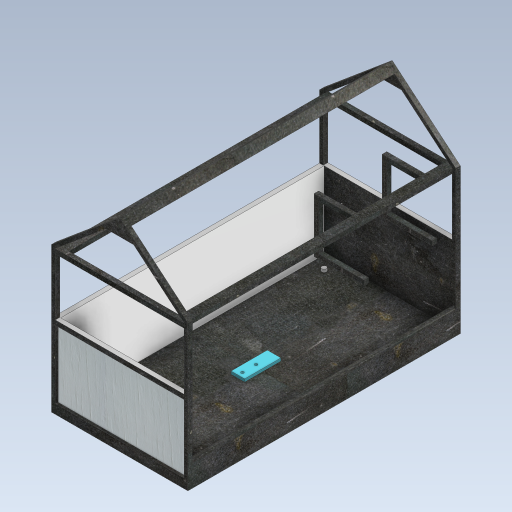
# Autodesk Inventor part: estructuragen
Saved by Autodesk Inventor 2023 (Build 270158000, 158)
## iProperties
Created: 2023-03-08
Part Number: estructuragen
Material: Steel
Document SubType Name: Modeling
Designer: santi
Density: 7.85 g/cm^3
Appearance: Plate
Author: santi
Autodesk Inventor part; units mm, degrees
ref_plane "YZ Plane" through (0, 0, 0) normal (1, 0, 0) x (0, 1, 0)
ref_plane "XZ Plane" through (0, 0, 0) normal (0, 1, 0) x (-1, 0, 0)
ref_plane "XY Plane" through (0, 0, 0) normal (0, 0, 1) x (1, 0, 0)
sketch "Sketch1" plane through (0, 0, 0) normal (0, 1, 0) x (-1, 0, 0)
  line L0 (0, 0) -> (150, 0)
  line L1 (150, 0) -> (150, -300)
  line L2 (150, -300) -> (0, -300)
  line L3 (0, -300) -> (0, 0)
  dimension "d0" = 150
  dimension "d1" = 300
  constraints: 8 end point, 2 parallel, 1 horizontal, 1 perpendicular
  measures "d0" distance of L1.end L2.end
  measures "d1" distance of L0.end L1.end
extrude "Extrusion1" add sketch "Sketch1" along normal blind 5
sketch "Sketch2" plane through (0, 5, 0) normal (0, 1, 0) x (1, 0, 0)
  line L0 (-150, 0) -> (0, 0) projected
  line L1 (0, 300) -> (-150, 300) projected
  line L2 (0, 0) -> (-150, 0)
  line L3 (-150, 0) -> (-150, 300)
  line L4 (-150, 300) -> (0, 300)
  line L5 (0, 300) -> (0, 0)
  line L6 (-145, 295) -> (-145, 5)
  line L7 (-145, 5) -> (-5, 5)
  line L8 (-5, 5) -> (-5, 295)
  line L9 (-5, 295) -> (-145, 295)
  line L10 (-5, 5) -> (-145, 5)
  line L11 (-145, 5) -> (-145, 295)
  line L12 (-145, 295) -> (-5, 295)
  line L13 (-5, 295) -> (-5, 5)
  line L14 (0, 0) -> (-150, 0)
  line L15 (-150, 0) -> (-150, 300)
  line L16 (-150, 300) -> (0, 300)
  line L17 (0, 300) -> (0, 0)
  point P0 (0, 300)
  point P1 (-150, 0)
  dimension "d4" = 5
  constraints: 32 end point, 8 parallel, 4 perpendicular, 3 horizontal, 3 other
  measures "d4" distance between parallel lines of L3 L6
extrude "Extrusion2" add sketch "Sketch2" along normal blind 5
sketch "Sketch3" plane through (-150, 0, 0) normal (0, 0, 1) x (1, 0, 0)
  line L0 (150, 10) -> (0, 10) projected
  line L1 (0, 10) -> (150, 10)
  line L2 (0, 10) -> (150, 10)
  line L3 (150, 10) -> (150, 160)
  line L4 (0, 10) -> (0, 160)
  line L5 (0, 160) -> (75, 222.9325)
  line L6 (75, 222.9325) -> (150, 160)
  line L7 (146, 10) -> (146, 158.1348)
  line L8 (146, 158.1348) -> (75, 217.7108)
  line L9 (75, 217.7108) -> (4, 158.1348)
  line L10 (4, 158.1348) -> (4, 10)
  line L11 (5, 10) -> (145, 10) projected
  line L12 (5, 10) -> (0, 10)
  line L13 (145, 10) -> (150, 10)
  point P0 (150, 0)
  dimension "d7" = 150
  dimension "d8" = 150
  dimension "d9" = 130
  dimension "d10" = 130
  dimension "d11" = 4
  constraints: 24 end point, 1 horizontal, 1 perpendicular, 1 vertical, 3 other
  measures "d7" distance of L0.start L3.end
  measures "d8" distance of L0.end L4.end
  measures "d9" angle of L4 L5
  measures "d10" angle of L6 L3
  measures "d11" distance between parallel lines of L6 L8
extrude "Extrusion3" add sketch "Sketch3" against normal blind 5 contours L0 L7 L8 L9 L10 L4 L5 L6 L3
ref_plane "Work Plane1" through (-150, 0, -150) normal (0, 0, 1) x (1, 0, 0)
mirror "Mirror1" about plane through (-150, 0, -150) normal (0, 0, 1) of "Extrusion3"
sketch "Sketch4" plane through (-150, 0, -5) normal (0, 0, -1) x (-1, 0, 0)
  line L0 (-145, 10) -> (-5, 10) projected
  line L1 (-5, 10) -> (-3, 10)
  line L2 (-3, 10) -> (-3, 90)
  line L3 (-3, 90) -> (-5, 90)
  line L4 (-5, 90) -> (-5, 10)
  point P0 (-150, 0)
  dimension "d14" = 2
  dimension "d15" = 80
  constraints: 8 end point, 2 parallel, 1 horizontal, 1 perpendicular
  measures "d14" distance of L3.end L2.end
  measures "d15" distance of L2.end L1.end
extrude "Extrusion4" add sketch "Sketch4" along normal up to surface (290 mm away)
sketch "Sketch5" plane through (-4, 10, -300) normal (-1, 0, 0) x (0, 0, 1)
  line L0 (5, 0) -> (5, 80) projected
  line L1 (5, 0) -> (3, 0)
  line L2 (3, 0) -> (3, 80)
  line L3 (3, 80) -> (5, 80)
  line L4 (5, 80) -> (5, 0)
  point P0 (300, -10)
  point P1 (5, 80)
  dimension "d18" = 2
  dimension "d40" = 80
  constraints: 8 end point, 2 parallel, 1 horizontal, 1 perpendicular
  measures "d18" distance of L2.end L3.end
  measures "d40" distance of L1.end L2.end
extrude "Extrusion5" add sketch "Sketch5" along normal up to surface (142 mm away)
mirror "Mirror2" about plane through (-150, 0, -150) normal (0, 0, 1) of "Extrusion5"
sketch "Sketch12" plane through (-146, 10, 0) normal (1, 0, 0) x (0, 0, -1)
  line L0 (3, 0) -> (3, 80) construction
  line L1 (3, 80) -> (3, 75)
  line L2 (3, 75) -> (0, 75)
  line L3 (0, 0) -> (0, 148.1348) construction
  line L4 (0, 75) -> (0, 80)
  line L5 (0, 80) -> (3, 80)
  point P0 (0, -10)
  dimension "d43" = 5
  constraints: 8 end point, 2 perpendicular, 2 point on line, 1 vertical
  measures "d43" distance of L0.end L1.end
extrude "Extrusion10" add sketch "Sketch12" along normal up to surface (142 mm away)
mirror "Mirror4" about plane through (-150, 0, -150) normal (0, 0, 1) of "Extrusion10"
sketch "Sketch13" plane through (-5, 5, -5) normal (0, 0, -1) x (-1, 0, 0)
  line L0 (141, 85) -> (-1, 85) construction
  line L1 (145, -5) -> (145, 155) construction
  line L2 (141, 85) -> (145, 85)
  line L3 (145, 85) -> (145, 80)
  line L4 (145, 80) -> (141, 80)
  line L5 (141, 80) -> (141, 85)
  point P0 (-5, -5)
  dimension "d46" = 5
  constraints: 8 end point, 2 parallel, 1 horizontal, 1 perpendicular, 1 point on line
  measures "d46" distance of L2.end L3.end
extrude "Extrusion11" add sketch "Sketch13" along normal up to surface (290 mm away)
chamfer "Chamfer1" distance 20 angle 45 1 edges at (-75, 217.7108, -297.5)
chamfer "Chamfer2" distance 20 angle 45 1 edges at (-75, 217.7108, -2.5)
sketch "Sketch16" plane through (-150, 0, 0) normal (0, 0, 1) x (1, 0, 0)
  circle A0 centre (75, 214.8551) radius 1.5
  line L0 (90.3209, 204.8551) -> (59.6791, 204.8551) projected
  point P0 (150, 0)
  point P1 (75, 204.8551)
  point P2 (75, 222.9325)
  dimension "d62" = 3
  dimension "d63" = 10
  constraints: 1 centre point, 1 midpoint, 1 vertical alignment
  measures "d62" diameter of A0
  measures "d63" distance of point (75, 204.855) A0.centre
extrude "Extrusion14" cut sketch "Sketch16" against normal blind 310.0375
sketch "Sketch17" plane through (-145, 5, -295) normal (0, 0, 1) x (1, 0, 0)
  line L0 (145, 155) -> (70, 217.9325) construction
  line L1 (70, 217.9325) -> (62.3396, 211.5046)
  line L2 (70, 217.9325) -> (-5, 155) construction
  line L3 (62.3396, 211.5046) -> (77.6604, 211.5046)
  line L4 (77.6604, 211.5046) -> (70, 217.9325)
  point P0 (145, -5)
  dimension "d70" = 10
  constraints: 6 end point, 2 point on line, 1 horizontal
  measures "d70" distance of L0.end L1.end
extrude "Extrusion15" add sketch "Sketch17" along normal up to surface (290 mm away)
sketch "Sketch19" plane through (-146, 158.1348, -295) normal (1, 0, 0) x (0, 0, -1)
  line L0 (5, 1.8652) -> (0, 1.8652) construction
  line L1 (0, 1.8652) -> (0, 58.3698) construction
  line L2 (0, 1.8652) -> (5, 1.8652) construction
  line L3 (0, 1.8652) -> (0, -0.1348) construction
  line L4 (0, -68.1348) -> (0, 1.8652) construction
  line L5 (0, -0.1348) -> (5, -0.1348) construction
  line L6 (5, -158.1348) -> (5, 1.8652) construction
  line L7 (5, 64.7977) -> (5, 1.8652) construction
  line L8 (5, -0.1348) -> (5, 1.8652) construction
  line L9 (0, -0.1348) -> (5, -0.1348)
  line L10 (5, -0.1348) -> (5, -5.1348)
  line L11 (5, -5.1348) -> (0, -5.1348)
  line L12 (0, -5.1348) -> (0, -0.1348)
  point P0 (-295, -158.1348)
  dimension "d77" = 2
  dimension "d78" = 5
  constraints: 16 end point, 3 point on line, 2 horizontal, 2 parallel, 2 perpendicular, 1 vertical
  measures "d77" distance of L0.end L3.end
  measures "d78" distance of L9.end L10.end
extrude "Extrusion17" add sketch "Sketch19" along normal up to surface (142 mm away)
mirror "Mirror5" about plane through (-150, 0, -150) normal (0, 0, 1) of "Extrusion17"
sketch "Sketch20" plane through (-5, 5, -5) normal (0, 0, -1) x (-1, 0, 0)
  line L0 (141, 153) -> (-1, 153) construction
  line L1 (141, 148) -> (-1, 148) construction
  line L2 (-1, 153) -> (9, 153)
  line L3 (9, 153) -> (9, 148)
  line L4 (9, 148) -> (-1, 148)
  line L5 (-1, 148) -> (-1, 153)
  line L6 (131, 148) -> (141, 148)
  line L7 (141, 148) -> (141, 153)
  line L8 (141, 153) -> (131, 153)
  line L9 (131, 153) -> (131, 148)
  point P0 (-5, -5)
  dimension "d81" = 10
  dimension "d84" = 10
  dimension "d85" = 142
  constraints: 16 end point, 4 parallel, 3 point on line, 2 horizontal, 2 perpendicular
  measures "d81" distance of L3.end L4.end
  measures "d84" distance of L8.end L7.end
  measures "d85" distance of L6.end L1.end
extrude "Extrusion18" add sketch "Sketch20" along normal up to surface (290 mm away)
sketch "Sketch21" plane through (-14, 153, -295) normal (-1, 0, 0) x (0, 0, 1)
  line L0 (290, 5) -> (0, 5) construction
  line L1 (290, 0) -> (0, 0) construction
  line L2 (20, 5) -> (25, 5)
  line L3 (25, 5) -> (25, 0)
  line L4 (25, 0) -> (20, 0)
  line L5 (20, 0) -> (20, 5)
  line L6 (95, 5) -> (100, 5)
  line L7 (100, 5) -> (100, 0)
  line L8 (100, 0) -> (95, 0)
  line L9 (95, 0) -> (95, 5)
  line L10 (0, 0) -> (290, 0) construction
  point P0 (295, -153)
  point P1 (145, 0)
  dimension "d86" = 5
  dimension "d87" = 5
  dimension "d88" = 80
  dimension "d96" = 20
  constraints: 18 end point, 5 parallel, 4 point on line, 2 horizontal, 2 perpendicular, 1 midpoint
  measures "d86" distance of L3.end L4.end
  measures "d87" distance of L7.end L8.end
  measures "d88" distance of L7.end L4.end
  measures "d96" distance of L4.end L1.end
extrude "Extrusion19" add sketch "Sketch21" along normal blind 42
sketch "Sketch22" plane through (-146, 153, 0) normal (0, -1, 0) x (1, 0, 0)
  line L0 (90, -195) -> (90, -200) projected
  line L1 (132, -200) -> (90, -200) construction
  line L2 (90, -195) -> (95, -195)
  line L3 (95, -195) -> (95, -200)
  line L4 (95, -200) -> (90, -200)
  line L5 (90, -200) -> (90, -195)
  line L6 (90, -270) -> (90, -275) projected
  line L7 (132, -275) -> (90, -275) construction
  line L8 (90, -270) -> (95, -270)
  line L9 (95, -270) -> (95, -275)
  line L10 (95, -275) -> (90, -275)
  line L11 (90, -275) -> (90, -270)
  point P0 (146, 0)
  dimension "d92" = 5
  dimension "d93" = 5
  constraints: 16 end point, 4 parallel, 2 horizontal, 2 perpendicular, 2 point on line
  measures "d92" distance of L3.end L4.end
  measures "d93" distance of L9.end L10.end
extrude "Extrusion20" add sketch "Sketch22" along normal blind 55
sketch "Sketch23" plane through (-51, 153, -195) normal (1, 0, 0) x (0, 0, -1)
  line L0 (0, 0) -> (0, -55) construction
  line L1 (5, 5) -> (5, -55) construction
  line L2 (0, -55) -> (5, -55)
  line L3 (5, -55) -> (5, -50)
  line L4 (5, -50) -> (0, -50)
  line L5 (0, -50) -> (0, -55)
  line L6 (75, 5) -> (75, -55) construction
  line L7 (80, 0) -> (80, -55) construction
  line L8 (75, -55) -> (80, -55)
  line L9 (80, -55) -> (80, -50)
  line L10 (80, -50) -> (75, -50)
  line L11 (75, -50) -> (75, -55)
  point P0 (-195, -153)
  dimension "d97" = 5
  constraints: 16 end point, 4 parallel, 3 point on line, 2 horizontal, 2 perpendicular
  measures "d97" distance of L3.end L2.end
extrude "Extrusion21" add sketch "Sketch23" along normal blind 50
sketch "Sketch24" plane through (0, 10, 0) normal (0, 1, 0) x (1, 0, 0)
  line L0 (-5, 5) -> (-5, 295) projected
  line L1 (0, 0) -> (0, 300) construction
  line L2 (-5, 5) -> (0, 5)
  line L3 (0, 5) -> (0, 295)
  line L4 (0, 295) -> (-5, 295)
  line L5 (-5, 295) -> (-5, 5)
  constraints: 8 end point, 2 parallel, 1 horizontal, 1 perpendicular, 1 point on line
extrude "Extrusion22" add sketch "Sketch24" along normal blind 16
sketch "Sketch26" plane through (-5, 5, -5) normal (0, 0, -1) x (-1, 0, 0)
  circle A0 centre (-2.5, 22) radius 1
  line L0 (-5, 21) -> (0, 21) construction
  point P0 (-5, -5)
  point P1 (-2.5, 21)
  dimension "d103" = 2
  constraints: 1 centre point, 1 midpoint, 1 tangent, 1 vertical alignment
  measures "d103" diameter of A0
extrude "Extrusion23" cut sketch "Sketch26" against normal blind 3
mirror "Mirror6" about plane through (-150, 0, -150) normal (0, 0, 1) of "Extrusion23"
fillet "Fillet1" radius 2 1 edges at (0, 26, -150)
sketch "Sketch27" plane through (0, 5, 0) normal (0, 1, 0) x (1, 0, 0)
  line L0 (-67.5, 130) -> (-82.5, 130)
  line L1 (-82.5, 130) -> (-82.5, 170)
  line L2 (-82.5, 170) -> (-67.5, 170)
  line L3 (-67.5, 170) -> (-67.5, 130)
  line L4 (-75, 300) -> (-75, 0) construction
  line L5 (-67.5, 130) -> (-82.5, 170) construction
  line L6 (-82.5, 130) -> (-67.5, 170) construction
  circle A0 centre (-75, 135) radius 1.5
  circle A1 centre (-75, 150) radius 1.5
  point P0 (0, 0)
  dimension "d107" = 15
  dimension "d108" = 40
  dimension "d111" = 3
  dimension "d112" = 3
  dimension "d113" = 15
  dimension "d114" = 5
  constraints: 12 end point, 4 midpoint, 2 centre point, 2 parallel, 1 horizontal, 1 perpendicular, 1 point on line
  measures "d107" distance of L1.end L2.end
  measures "d108" distance of L0.end L1.end
  measures "d111" diameter of A0
  measures "d112" diameter of A1
  measures "d113" distance of A1.centre A0.centre
  measures "d114" distance from line of L0 A0.centre
extrude "Extrusion24" add sketch "Sketch27" along normal blind 3
sketch "Sketch28" plane through (0, 5, 0) normal (0, 1, 0) x (1, 0, 0)
  circle A0 centre (-20, 20) radius 2.5
  line L0 (0, 0) -> (0, 300) construction
  line L1 (-150, 0) -> (0, 0) construction
  line L2 (-150, 300) -> (-150, 0) construction
  line L3 (-150, 150) -> (0, 150) construction
  line L4 (-75, 0) -> (-75, 300) construction
  line L5 (0, 300) -> (-150, 300) construction
  circle A1 centre (-20, 280) radius 2.5
  circle A2 centre (-130, 20) radius 2.5
  circle A3 centre (-130, 280) radius 2.5
  dimension "d115" = 5
  dimension "d116" = 20
  dimension "d117" = 20
  constraints: 4 centre point, 4 end point, 4 midpoint, 3 symmetric about line, 3 other
  measures "d115" diameter of A0
  measures "d116" distance from line of A0.centre L0
  measures "d117" distance from line of L1 A0.centre
extrude "Extrusion25" add sketch "Sketch28" along normal blind 3
body "Solid1"
